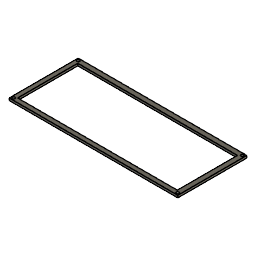
KeyboardBezel (Autodesk Fusion 360 design; units mm, degrees)
part number: 2026-01-27-16-23-20-670
Autodesk Fusion 360 part; units mm, degrees
sketch "Sketch1" plane through (0, 0, 0) normal (0, 0, 1) x (1, 0, 0)
  line L0 (0, 0) -> (-371, 0)
  line L1 (-371, 0) -> (-371, 152)
  line L2 (-371, 152) -> (0, 152)
  line L3 (0, 152) -> (0, 0)
  circle A0 centre (-366, 147) radius 1.7
  circle A1 centre (-5, 5) radius 1.7
  circle A2 centre (-366, 5) radius 1.7
  circle A3 centre (-5, 147) radius 1.7
  circle A4 centre (-366, 147) radius 3
  circle A5 centre (-5, 5) radius 3
  circle A6 centre (-366, 5) radius 3
  circle A7 centre (-5, 147) radius 3
  dimension "d1" = 371
  dimension "d2" = 152
  dimension "d3" = 3.4
  dimension "d4" = 5
  dimension "d5" = 5
  dimension "d6" = 3.4
  dimension "d7" = 3.4
  dimension "d8" = 3.4
  dimension "d9" = 5
  dimension "d10" = 5
  dimension "d11" = 5
  dimension "d12" = 5
  dimension "d13" = 5
  dimension "d14" = 5
  dimension "d15" = 6
  dimension "d16" = 6
  dimension "d17" = 6
  dimension "d18" = 6
  constraint horizontal L0
  constraint vertical L1
  constraint horizontal L2
  constraint vertical L3
  constraint coincident L0.start L3.end
  constraint coincident A1.centre A5.centre
  constraint coincident A3.centre A7.centre
  constraint coincident A0.centre A4.centre
  constraint coincident A2.centre A6.centre
  measures "d1" distance of L0.start L0.end
  measures "d2" distance of L0.start L2.end
  measures "d3" diameter of A0
  measures "d4" distance of L2 A0.centre
  measures "d5" distance of L1 A0.centre
  measures "d6" diameter of A1
  measures "d7" diameter of A2
  measures "d8" diameter of A3
  measures "d9" distance of L0 A2.centre
  measures "d10" distance of L1 A2.centre
  measures "d11" distance of L0 A1.centre
  measures "d12" distance of L3 A1.centre
  measures "d13" distance of L2 A3.centre
  measures "d14" distance of L3 A3.centre
  measures "d15" diameter of A4
  measures "d16" diameter of A5
  measures "d17" diameter of A6
  measures "d18" diameter of A7
sketch "Sketch2" plane through (0, 0, 0) normal (0, 0, 1) x (1, 0, 0)
  line L0 (-361.5, 141.5) -> (-10.5, 141.5)
  line L1 (-10.5, 141.5) -> (-10.5, 9.5)
  line L2 (-10.5, 9.5) -> (-361.5, 9.5)
  line L3 (-361.5, 9.5) -> (-361.5, 141.5)
  line L4 (0, 0) -> (-371, 0)
  line L5 (-371, 0) -> (-371, 152)
  dimension "d19" = 351
  dimension "d20" = 132
  dimension "d21" = 9.5
  dimension "d22" = 9.5
  constraint horizontal L0
  constraint vertical L1
  constraint horizontal L2
  constraint vertical L3
  measures "d19" distance of L0.start L0.end
  measures "d20" distance of L0.start L2.end
  measures "d21" distance of L2 L4
  measures "d22" distance of L3 L5
extrude "Extrude1" add sketch "Sketch1" along normal blind 5 contours L0 L1 L2 L3
extrude "Extrude2" cut sketch "Sketch2" along normal blind 10
